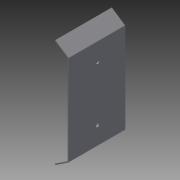
# Autodesk Inventor part: podpera_deska_rameno
Saved by Autodesk Inventor 2015 (Build 190159000, 159)
## iProperties
Created: 2015-03-15
Part Number: podpera_deska_rameno
Material: Generic
Document SubType Name: Modeling
Designer: Turboslimak
Density: 1 g/cm^3
Appearance: Default
Author: Turboslimak
Autodesk Inventor part; units mm, degrees
ref_plane "YZ Plane" through (0, 0, 0) normal (1, 0, 0) x (0, 1, 0)
ref_plane "XZ Plane" through (0, 0, 0) normal (0, 1, 0) x (-1, 0, 0)
ref_plane "XY Plane" through (0, 0, 0) normal (0, 0, 1) x (1, 0, 0)
sketch "Sketch1" plane through (0, 0, 0) normal (0, 1, 0) x (-1, 0, 0)
  line L0 (0.5, 41) -> (12.5, 49)
  line L1 (0.5, 41) -> (12.5, 49)
  line L2 (12.5, 49) -> (11.9453, 49.8321)
  line L3 (11.9453, 49.8321) -> (-0.0547, 41.8321)
  arc A0 (-0.0547, 41.8321) -> (-0.5, 41) centre (0.5, 41) ccw
  line L4 (0.5, 41) -> (0.5, 0)
  line L5 (0.5, 0) -> (-0.5, 0)
  line L6 (-0.5, 0) -> (-0.5, 41)
  line L7 (0.5, -41) -> (12.5, -49)
  line L8 (12.5, -49) -> (11.9453, -49.8321)
  line L9 (11.9453, -49.8321) -> (-0.0547, -41.8321)
  arc A1 (-0.5, -41) -> (-0.0547, -41.8321) centre (0.5, -41) ccw
  line L10 (0.5, -41) -> (0.5, 0)
  line L11 (-0.5, 0) -> (-0.5, -41)
  point P0 (0, 0)
  dimension "d0" = 1
  dimension "d4" = 1
  constraints: 24 end point, 6 symmetric about line, 4 point on circle, 2 centre point, 2 equal length, 2 perpendicular, 1 tangent, 1 other
  measures "d0" distance of L6.end L0.start
  measures "d4" distance of L2.end L0.end
extrude "Extrusion1" add sketch "Sketch1" along normal blind 52
sketch "Sketch2" plane through (-0.5, 0, -41) normal (-1, 0, 0) x (0, 0, 1)
  circle A0 centre (15.8425, 26.5) radius 1.5
  circle A1 centre (66.1575, 26.5) radius 1.5
  dimension "d10" = 3
  dimension "d11" = 3
  constraints: 2 centre point
  measures "d10" diameter of A0
  measures "d11" diameter of A1
extrude "Extrusion2" cut sketch "Sketch2" against normal blind 1
body "Solid1"
